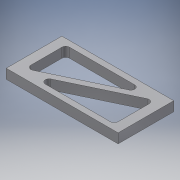
# Autodesk Inventor part: リンク_ふくらはぎ_サブフレーム_1_2(予備案)
Saved by Autodesk Inventor 2018 (Build 220112000, 112)
## iProperties
Created: 2016-06-03
Part Number: リンク_ふくらはぎ_サブフレーム_1_2(予備案)
Material: アルミニウム 2014-T4
Document SubType Name: Modeling
Designer: hiroaki
Density: 2.8 g/cm^3
Appearance: サテン
Mass: 10.4768 g
Surface Area: 35.4603 cm^2
Volume: 3.74171 cm^3
Author: hiroaki
Autodesk Inventor part; units mm, degrees
ref_plane "YZ Plane" through (0, 0, 0) normal (1, 0, 0) x (0, 1, 0)
ref_plane "XZ Plane" through (0, 0, 0) normal (0, 1, 0) x (-1, 0, 0)
ref_plane "XY Plane" through (0, 0, 0) normal (0, 0, 1) x (1, 0, 0)
sketch "スケッチ1" plane through (0, 0, 0) normal (0, 0, 1) x (1, 0, 0)
  line L0 (-29.15, 14.5) -> (29.15, 14.5)
  line L1 (29.15, 14.5) -> (29.15, -14.5)
  line L2 (29.15, -14.5) -> (-29.15, -14.5)
  line L3 (-29.15, -14.5) -> (-29.15, 14.5)
  line L4 (-24.15, 11.5) -> (24.15, 11.5) construction
  line L5 (24.15, 11.5) -> (24.15, -11.5) construction
  line L6 (24.15, -11.5) -> (-24.15, -11.5) construction
  line L7 (-24.15, -11.5) -> (-24.15, 11.5) construction
  line L8 (24.15, 11.5) -> (-24.15, -11.5) construction
  line L9 (-24.15, -9.8386) -> (-24.15, 11.5)
  line L10 (-24.15, 11.5) -> (20.6611, 11.5)
  line L11 (20.6611, 11.5) -> (-24.15, -9.8386)
  line L12 (-20.6611, -11.5) -> (24.15, -11.5)
  line L13 (24.15, -11.5) -> (24.15, 9.8386)
  line L14 (24.15, 9.8386) -> (-20.6611, -11.5)
  line L15 (-29.15, 12) -> (29.15, 12) construction
  line L16 (29.15, -12) -> (-29.15, -12) construction
  line L17 (29.15, 12) -> (29.15, -12) construction
  point P0 (0, 0)
  point P1 (0, 11.5)
  point P2 (0, 14.5)
  point P3 (24.15, 0)
  point P4 (29.15, 0)
  dimension "d0" = 5
  dimension "d1" = 3
  dimension "d2" = 1.5
  dimension "d3" = 24
  dimension "d4" = 2.5
  dimension "d16" = 58.3
  constraints: 36 end point, 6 parallel, 5 collinear, 5 horizontal, 5 midpoint, 4 perpendicular, 4 point on line, 2 horizontal alignment, 2 vertical alignment, 1 vertical, 1 other
  measures "d0" distance between parallel lines of L3 L7
  measures "d1" distance between parallel lines of L0 L4
  measures "d2" distance between parallel lines of L8 L11
  measures "d3" distance between parallel lines of L16 L15
  measures "d4" distance between parallel lines of L2 L16
  measures "d16" distance of L0.start L0.end
extrude "押し出し1" add sketch "スケッチ1" along normal blind 5
fillet "フィレット1" radius 2 6 edges at (-20.6611, -11.5, 2.5) (-24.15, -9.8386, 2.5) (24.15, 9.8386, 2.5) (24.15, -11.5, 2.5) (-24.15, 11.5, 2.5) (20.6611, 11.5, 2.5)
equation "\"d3\" = d5_1"
equation "\"d5_1\" = 24"
